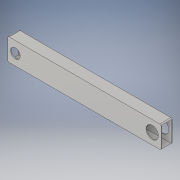
# Autodesk Inventor part: SideBar13v2
Saved by Autodesk Inventor 2018.3 (Build 223284000, 284)
## iProperties
Created: 2020-01-25
Part Number: SideBar13v2
Material: Aluminum 6061
Document SubType Name: Modeling
Designer: Myers
Mass: 209.157 g
Surface Area: 989.05 cm^2
Volume: 77.4655 cm^3
Density: 2.7 g/cm^3
Appearance: Aluminum - Dark
Author: Myers
Autodesk Inventor part; units mm, degrees
ref_plane "YZ Plane" through (0, 0, 0) normal (1, 0, 0) x (0, 1, 0)
ref_plane "XZ Plane" through (0, 0, 0) normal (0, 1, 0) x (-1, 0, 0)
ref_plane "XY Plane" through (0, 0, 0) normal (0, 0, 1) x (1, 0, 0)
sketch "Sketch1" plane through (0, 0, 0) normal (0, 0, 1) x (1, 0, 0)
  line L0 (-173.3804, -25.4) -> (173.3804, -25.4)
  line L1 (176.5554, -22.225) -> (176.5554, 22.225)
  line L2 (173.3804, 25.4) -> (-173.3804, 25.4)
  line L3 (-176.5554, 22.225) -> (-176.5554, -22.225)
  circle A0 centre (-159.0929, 0) radius 11.1125
  circle A1 centre (155.9179, 0) radius 14.2875
  arc A2 (-176.5554, -22.225) -> (-173.3804, -25.4) centre (-173.3804, -22.225) ccw
  arc A3 (173.3804, -25.4) -> (176.5554, -22.225) centre (173.3804, -22.225) ccw
  arc A4 (176.5554, 22.225) -> (173.3804, 25.4) centre (173.3804, 22.225) ccw
  arc A5 (-173.3804, 25.4) -> (-176.5554, 22.225) centre (-173.3804, 22.225) ccw
  point P0 (0, 0)
  point P1 (-176.5554, -25.4)
  point P2 (176.5554, 25.4)
  point P3 (176.5554, -25.4)
  point P4 (-176.5554, 25.4)
  point P5 (-176.5554, 0)
  point P6 (0, 25.4)
  dimension "d5" = 315.0108
  dimension "d6" = 22.225
  dimension "d7" = 20.6375
  dimension "d8" = 17.4625
  dimension "d9" = 50.8
  dimension "d11" = 3.175
  dimension "d16" = 28.575
  constraints: 8 end point, 8 point on circle, 8 point on line, 8 tangent, 6 centre point, 3 equal radius, 3 horizontal alignment, 2 midpoint, 2 parallel, 1 horizontal, 1 perpendicular, 1 vertical alignment
  measures "d5" distance of A1.centre A0.centre
  measures "d6" diameter of A0
  measures "d7" distance from line of L1 A1.centre
  measures "d8" distance from line of A0.centre L3
  measures "d9" distance of point (176.555, -25.4) point (176.555, 25.4)
  measures "d11" radius of A5
  measures "d16" diameter of A1
extrude "Extrusion1" add sketch "Sketch1" along normal blind 25.4
sketch "Sketch2" plane through (0, 0, 0) normal (1, 0, 0) x (0, 1, 0)
  line L0 (25.4, 25.4) -> (22.225, 25.4) projected
  line L1 (-22.225, 25.4) -> (22.225, 25.4) projected
  line L2 (-22.225, 25.4) -> (-25.4, 25.4) projected
  line L3 (-25.4, 0) -> (-25.4, 25.4) projected
  line L4 (-22.225, 0) -> (-25.4, 0) projected
  line L5 (-22.225, 0) -> (22.225, 0) projected
  line L6 (25.4, 0) -> (22.225, 0) projected
  line L7 (25.4, 0) -> (25.4, 25.4) projected
  line L8 (23.8125, 23.8125) -> (6.35, 23.8125)
  line L9 (6.35, 23.8125) -> (-6.35, 23.8125)
  line L10 (-6.35, 23.8125) -> (-23.8125, 23.8125)
  line L11 (-23.8125, 23.8125) -> (-23.8125, 1.5875)
  line L12 (-23.8125, 1.5875) -> (-6.35, 1.5875)
  line L13 (-6.35, 1.5875) -> (6.35, 1.5875)
  line L14 (6.35, 1.5875) -> (23.8125, 1.5875)
  line L15 (23.8125, 1.5875) -> (23.8125, 23.8125)
  dimension "d15" = 1.5875
  constraints: 16 end point, 7 other
  measures "d15" distance between parallel lines of L7 L15
extrude "Extrusion2" cut sketch "Sketch2" along normal through all both and the other way through all contours L15 L14 L13 L12 L11 L10 L9 L8
body "Solid1"
